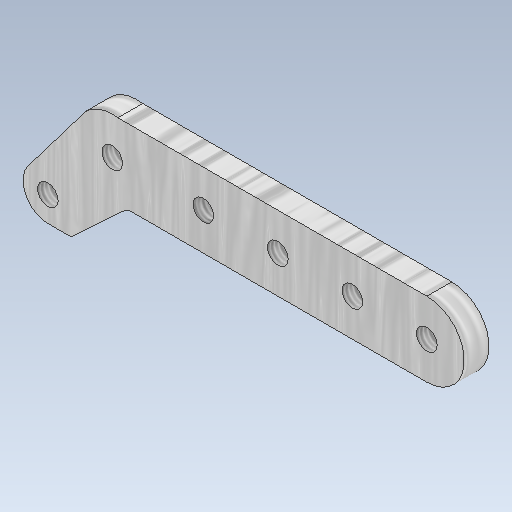
# Autodesk Inventor part: 中間節アーム先端締結パーツ外
Saved by Autodesk Inventor 2020.2 (Build 242310000, 310)
## iProperties
Created: 2020-03-28
Part Number: 中間節アーム先端締結パーツ外
Material: アルミニウム 7075
Document SubType Name: Modeling
Designer: aoyam
Density: 2.81 g/cm^3
Appearance: サテン - ブラシ仕上げ 重厚
Mass: 4.46679 g
Surface Area: 16.9082 cm^2
Volume: 1.5896 cm^3
Author: aoyam
Autodesk Inventor part; units mm, degrees
ref_plane "YZ Plane" through (0, 0, 0) normal (1, 0, 0) x (0, 1, 0)
ref_plane "XZ Plane" through (0, 0, 0) normal (0, 1, 0) x (-1, 0, 0)
ref_plane "XY Plane" through (0, 0, 0) normal (0, 0, 1) x (1, 0, 0)
sketch "スケッチ1" plane through (0, 0, 0) normal (0, 0, 1) x (1, 0, 0)
  circle A0 centre (-55, 0) radius 8.025 construction
  circle A1 centre (0, 0) radius 1.25 construction
  arc A2 (-44.5788, 6) -> (-63.6661, 8.3366) centre (-55, 0) ccw construction
  line L0 (-63.6661, 8.3366) -> (-109.1623, -38.9576) construction
  line L1 (-102.7709, -46.5745) -> (-48.2949, -9.9821) construction
  arc A3 (-48.2949, -9.9821) -> (-44.5788, -6) centre (-55, 0) ccw construction
  line L2 (-44.5788, -6) -> (-5.2915, -6) construction
  arc A4 (-5.2915, -6) -> (-5.2915, 6) centre (0, 0) ccw construction
  line L3 (-5.2915, 6) -> (-44.5788, 6) construction
  circle A5 centre (0, 0) radius 1.25
  circle A6 centre (-30, 0) radius 1.25
  circle A7 centre (-12, 0) radius 1.25
  circle A8 centre (-21, 0) radius 1.25
  line L4 (-30, 0) -> (0, 0)
  line L5 (-30, 0) -> (-50, 0)
  line L6 (-50, 0) -> (-30, 0)
  circle A9 centre (-50, 0) radius 1.25
  circle A10 centre (-50, 0) radius 4.025 construction
  circle A11 centre (-50, 0) radius 7.125 construction
  circle A12 centre (-57.7782, -7.7782) radius 1.25
  circle A13 centre (-57.7782, -7.7782) radius 3 construction
  line L7 (-50, 0) -> (-57.7782, -7.7782) construction
  line L8 (-53.1753, 3.2604) -> (-60.169, -5.9659)
  line L9 (-55.3874, -9.5904) -> (-46.209, 2.5181)
  arc A14 (-46.209, 2.5181) -> (-53.1753, 3.2604) centre (-50, 0) ccw
  arc A15 (-60.169, -5.9659) -> (-55.3874, -9.5904) centre (-57.7782, -7.7782) ccw
  line L10 (-50, 0) -> (0, 0) construction
  line L11 (-50, -4.5) -> (0, -4.5)
  line L12 (0, 4.5) -> (-50, 4.5)
  arc A16 (-50, 4.5) -> (-50, -4.5) centre (-50, 0) ccw
  arc A17 (0, -4.5) -> (0, 4.5) centre (0, 0) ccw
  line L13 (-57.7782, -10.7782) -> (-54.9706, -10.7782)
  line L14 (-54.9706, -10.7782) -> (-48.1997, -4.5)
  line L15 (-50, 0) -> (-57.7782, -7.7782)
  circle A18 centre (-12, 0) radius 4.5
  point P0 (-53.8891, -3.8891)
  point P1 (-25, 0)
  point P2 (-48.7574, -3)
  point P3 (-49.3198, 4.5)
  point P4 (-53.5862, 2.7184)
  point P5 (-51.3675, -4.2872)
  point P6 (-12, -4.5)
  point P7 (-12, 4.5)
  dimension "d0" = 20
  dimension "d2" = 2.5
  dimension "d3" = 8.05
  dimension "d4" = 3.1
  dimension "d5" = 30
  dimension "d6" = 2.5
  dimension "d7" = 2.5
  dimension "d8" = 2.5
  dimension "d9" = 2.5
  dimension "d11" = 9
  dimension "d13" = 2.5
  dimension "d14" = 6
  dimension "d15" = 6
  dimension "d16" = 9
  dimension "d21" = 135
  dimension "d22" = 10
  dimension "d30" = 9
  dimension "d31" = 11
  constraints: 36 end point, 19 centre point, 15 point on circle, 8 tangent, 5 coincident, 4 horizontal, 2 midpoint, 2 parallel, 2 point on line, 1 collinear, 22 other
  measures "d0" distance of L4.start L5.end
  measures "d2" diameter of A9
  measures "d3" diameter of A10
  measures "d4" radial gap between concentric circles of A10 A11
  measures "d5" distance of L4.start L4.end
  measures "d6" diameter of A5
  measures "d7" diameter of A7
  measures "d8" diameter of A8
  measures "d9" diameter of A6
  measures "d11" distance of A7.centre A8.centre
  measures "d13" diameter of A12
  measures "d14" diameter of A13
  measures "d15" diameter of A15
  measures "d16" diameter of A17
  measures "d21" angle of L10 L7
  measures "d22" angle of L9 L14
  measures "d30" distance of L4.start A8.centre
  measures "d31" distance of A12.centre L5.end
extrude "押し出し1" add sketch "スケッチ1" along normal blind 3 contours L4 A8 A18 L11 A16 L9 L5 A6 | A6 L5 L9 A14 L12 A18 L4 A8 | L9 A16 L15 A9 L5 | L5 A9 L15 A16 L12 A14 L9 | A16 L11 L14 L13 A15 L9 | L9 A15 L8 A16 | A18 L4 A7 | L4 A7 A18 | L12 A16 L8 A14
fillet "フィレット1" radius 1.05 1 edges at (-48.1997, -4.5, 1.5)
sketch "スケッチ2" plane through (0, 0, 3) normal (0, 0, 1) x (1, 0, 0)
  arc A0 (-60.7927, -6.5251) -> (-59.7797, -5.8711) centre (-60.7525, -5.4759) ccw
  arc A1 (-55.3849, -4.4725) -> (-59.7797, -5.8711) centre (-57.0004, -7.0004) ccw
  arc A2 (-55.3849, -4.4725) -> (-43.7567, 3.1657) centre (-50, 0) ccw
  arc A3 (-44.0452, 4.6286) -> (-43.7567, 3.1657) centre (-43.1001, 4.055) ccw
  line L0 (-44.0452, 4.6286) -> (-41.5381, 8.9709)
  arc A4 (-41.5381, 8.9709) -> (-46.5567, 11.6351) centre (-44, 10.3923) ccw
  line L1 (-46.5567, 11.6351) -> (-49.0637, 7.2927)
  arc A5 (-50.5985, 6.9744) -> (-49.0637, 7.2927) centre (-49.9731, 7.8177) ccw
  arc A6 (-50.5985, 6.9744) -> (-50.2678, 6.9949) centre (-50, 0) ccw
  circle A7 centre (-50, 0) radius 4.025
  circle A8 centre (-50, 0) radius 1.25 projected
  circle A9 centre (-39, 0) radius 4
  line L2 (-50, 0) -> (-38.3804, 0)
  circle A10 centre (-39, 0) radius 1.25
  circle A11 centre (-30, 0) radius 1.25 projected
  point P0 (0, 0)
  point P1 (-43.3711, 2.3255)
  point P2 (-43, 0)
  point P3 (-49.3534, 6.9701)
  point P4 (-44.1966, 3.9141)
  point P5 (-43.7567, 3.1657)
  dimension "d23" = 12
  dimension "d24" = 8
  dimension "d27" = 2.5
  dimension "d28" = 9
  dimension "d29" = 7
  constraints: 14 point on circle, 10 centre point, 6 end point, 3 coincident, 2 concentric, 2 tangent, 1 horizontal, 1 point on line
  measures "d23" distance of A4.centre point (-50, 0)
  measures "d24" diameter of A9
  measures "d27" diameter of A10
  measures "d28" distance of A11.centre A9.centre
  measures "d29" radius of A6
extrude "押し出し2" cut sketch "スケッチ2" against normal blind 3 contours A10
thread "ねじ1" size "M3x0.5" class "6H" standard "ANSI Metric M Profile" full length
thread "ねじ2" size "M3x0.5" class "6H" standard "ANSI Metric M Profile" full length
thread "ねじ3" size "M3x0.5" class "6H" standard "ANSI Metric M Profile" full length
thread "ねじ4" size "M3x0.5" class "6H" standard "ANSI Metric M Profile" full length
thread "ねじ5" size "M3x0.5" class "6H" standard "ANSI Metric M Profile" full length
thread "ねじ6" size "M3x0.5" class "6H" standard "ANSI Metric M Profile" full length
